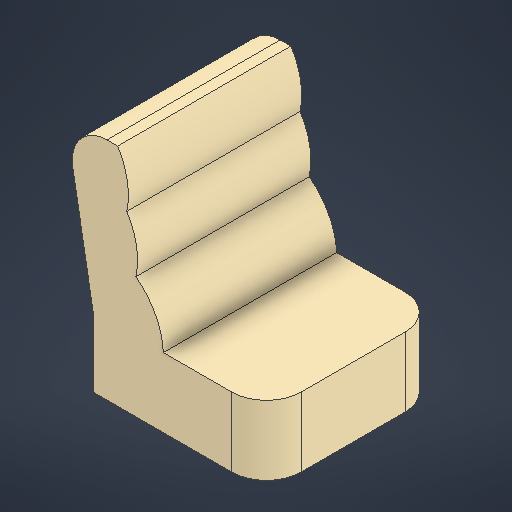
# Autodesk Inventor part: fotel
Saved by Autodesk Inventor 2026.2 (Build 302298000, 298)
## iProperties
Created: 2026-08-18
Part Number: fotel
Material: Tworzywo sztuczne ABS
Document SubType Name: Modeling
Designer: wojsl
Density: 1.06 g/cm^3
Appearance: Gładki — biały
Author: wojsl
Autodesk Inventor part; units mm, degrees
ref_plane "YZ Plane" through (0, 0, 0) normal (1, 0, 0) x (0, 1, 0)
ref_plane "XZ Plane" through (0, 0, 0) normal (0, 1, 0) x (-1, 0, 0)
ref_plane "XY Plane" through (0, 0, 0) normal (0, 0, 1) x (1, 0, 0)
sketch "Szkic1" plane through (0, 0, 0) normal (0, 1, 0) x (-1, 0, 0)
  line L0 (-2.4857, -2.5762) -> (1.5143, -2.5762)
  line L1 (1.5143, -2.5762) -> (1.5143, 2.4238)
  line L2 (1.5143, 2.4238) -> (-2.4857, 2.4238)
  line L3 (-3.4857, 1.4238) -> (-3.4857, -1.5762)
  arc A0 (-2.4857, 2.4238) -> (-3.4857, 1.4238) centre (-2.4857, 1.4238) ccw
  arc A1 (-3.4857, -1.5762) -> (-2.4857, -2.5762) centre (-2.4857, -1.5762) ccw
  point P0 (0, 0)
  point P1 (-3.4857, 2.4238)
  dimension "d0" = 5
  dimension "d1" = 5
  dimension "d2" = 1
  constraints: 8 end point, 4 point on circle, 4 tangent, 2 centre point, 2 parallel, 2 point on line, 1 equal radius, 1 horizontal, 1 perpendicular
  measures "d0" distance of L0.end L1.end
  measures "d1" distance of L1.end point (-3.486, 2.424)
  measures "d2" radius of A0
extrude "Wyciągnięcie proste1" add sketch "Szkic1" along normal blind 2
sketch "Szkic2" plane through (0, 0, 0) normal (0, -1, 0) x (1, 0, 0)
  circle A0 centre (0.3828, -1.0762) radius 0.5
  circle A1 centre (0.3828, 0.9238) radius 0.5
  line L0 (2.4857, -2.5762) -> (-1.5143, -2.5762) projected
  line L1 (-1.5143, 2.4238) -> (2.4857, 2.4238) projected
  point P0 (0, 0)
  dimension "d5" = 1
  dimension "d6" = 1
  dimension "d7" = 2
  dimension "d8" = 1
  dimension "d9" = 1.5
  dimension "d10" = 1.5
  constraints: 2 centre point
  measures "d5" diameter of A0
  measures "d6" diameter of A1
  measures "d7" distance of A1.centre A0.centre
  measures "d8" distance of A1.centre point (0, 0)
  measures "d9" distance from line of A0.centre L0
  measures "d10" distance from line of L1 A1.centre
extrude "Wyciągnięcie proste2" cut sketch "Szkic2" against normal blind 1
sketch "Szkic3" plane through (2.4857, 0, -2.5762) normal (0, 0, -1) x (-1, 0, 0)
  line L0 (0, 2) -> (4, 2) projected
  line L1 (4, 2) -> (4.2645, 3.5)
  line L2 (4.2645, 3.5) -> (2.7645, 3.5)
  line L3 (1.9737, 2) -> (4, 2)
  arc A0 (2.7645, 3.5) -> (1.9737, 2) centre (3.9714, 1.9052) ccw
  line L4 (4, 2) -> (4.7935, 6.5)
  line L5 (4.529, 5) -> (3.029, 5)
  arc A1 (3.029, 5) -> (2.7645, 3.5) centre (4.718, 3.9289) ccw
  line L6 (4.7935, 6.5) -> (3.2935, 6.5)
  arc A2 (3.2935, 6.5) -> (3.029, 5) centre (4.9825, 5.4289) ccw
  point P0 (2.4857, 0)
  point P1 (2, 2)
  point P2 (1.9737, 2)
  point P3 (3.5145, 3.5)
  dimension "d15" = 100
  dimension "d16" = 1.5
  dimension "d17" = 2
  dimension "d18" = 0
  dimension "d24" = 1.5
  dimension "d28" = 1.5
  dimension "d29" = 100
  dimension "d30" = 1.5
  dimension "d31" = 2
  dimension "d32" = 1.5
  dimension "d33" = 1.5
  dimension "d34" = 2
  constraints: 12 end point, 6 point on circle, 3 centre point, 2 midpoint, 2 parallel, 1 horizontal, 1 point on line
  measures "d15" angle of L0 L1
  measures "d16" distance of L1.end L2.end
  measures "d17" radius of A0
  measures "d18" vertical distance of point (2, 2) L3.start
  measures "d24" distance between parallel lines of L0 L2
  measures "d28" distance from line of point (3.514, 3.5) L5
  measures "d29" angle of L0 L4
  measures "d30" distance of L5.start L5.end
  measures "d31" radius of A1
  measures "d32" distance of L4.end L6.end
  measures "d33" distance between parallel lines of L5 L6
  measures "d34" radius of A2
extrude "Wyciągnięcie proste3" add sketch "Szkic3" against normal blind 5 contours A0 L2 L1 L0
extrude "Wyciągnięcie proste4" add sketch "Szkic3" against normal blind 5 contours A1 L5 L4 L2 | A2 L6 L4 L5
fillet "Zaokrąglenie1" radius 1 1 edges at (-2.3078, 6.5, -0.0762)
